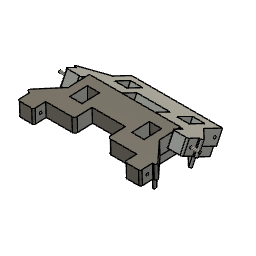
trackcomponent (Autodesk Fusion 360 design; units mm, degrees)
Autodesk Fusion 360 part; units mm, degrees
note: some values were not read from the file. Set by a fixed rule: which sketch regions a step uses.
sketch "Sketch1" plane through (0, 0, 0) normal (0, 0, 1) x (1, 0, 0)
  line L0 (0, 0) -> (0, -49.8745) construction
  line L1 (-9.5, 0) -> (-26, 0)
  line L2 (-35, 0) -> (-35, -7)
  line L3 (-35, -7) -> (-26, -7)
  line L4 (-26, -7) -> (-26, 0)
  line L5 (0, 0) -> (0, 25)
  line L6 (0, 25) -> (-26, 25)
  line L7 (-26, 25) -> (-26, 13)
  line L8 (-35, 0) -> (-38, 0)
  line L9 (-38, 0) -> (-26, 13)
  line L10 (-9.5, 0) -> (-9.5, 10)
  line L11 (-9.5, 10) -> (0, 10)
  line L12 (-21.25, 19.0231) -> (-14.25, 19.0231)
  line L13 (-14.25, 19.0231) -> (-14.25, 9.0231)
  line L14 (-14.25, 9.0231) -> (-21.25, 9.0231)
  line L15 (-21.25, 9.0231) -> (-21.25, 19.0231)
  line L16 (-36.7752, 0) -> (-25.1001, 12.6481)
  line L17 (-25.1001, 24.3) -> (-25.1001, 12.6481)
  line L18 (0, 24.3) -> (-25.1001, 24.3)
  line L19 (-34.7338, 0) -> (-23.6001, 12.0616)
  line L20 (-23.6001, 22.8) -> (-23.6001, 12.0616)
  line L21 (0, 22.8) -> (-23.6001, 22.8)
  line L22 (-34.7338, 0) -> (-35, 0)
  dimension "d1" = 35
  dimension "d3" = 9
  dimension "d8" = 7
  dimension "d10" = 25
  dimension "d12" = 3
  dimension "d13" = 10
  dimension "d14" = 10
  dimension "d15" = 7
  dimension "d19" = 12
  dimension "d20" = 9.5
  dimension "d21" = 16.5
  dimension "d22" = 4.75
  dimension "d41" = 1.5
  dimension "d42" = 1.5
  dimension "d43" = 1.5
  dimension "d44" = 0.7
  constraint vertical L0
  constraint perpendicular L0 L1
  constraint perpendicular L1 L2
  constraint perpendicular L2 L3
  constraint perpendicular L1 L4
  constraint perpendicular L1 L5
  constraint perpendicular L4 L6
  constraint perpendicular L6 L7
  constraint perpendicular L2 L8
  constraint coincident L5 L11.end
  constraint perpendicular L5 L11
  constraint horizontal L12
  constraint vertical L13
  constraint horizontal L14
  constraint vertical L15
  constraint parallel L9 L19
  constraint parallel L7 L20
  constraint parallel L6 L21
  constraint coincident L8 L19.start
  constraint parallel L9 L16
  constraint parallel L7 L17
  constraint parallel L6 L18
  constraint coincident L8 L16.start
  constraint perpendicular L2 L22
  measures "d1" distance of L0.start L2.start
  measures "d3" distance of L2.end L3.end
  measures "d8" distance of L2.start L2.end
  measures "d10" distance of L0.start L5.end
  measures "d12" distance of L2.start L8.end
  measures "d13" distance of L1.start L10.end
  measures "d14" distance of L12.start L14.end
  measures "d15" distance of L12.start L12.end
  measures "d19" distance of L6.end L7.end
  measures "d20" distance of L10.end L11.end
  measures "d21" horizontal distance of L7.end L10.end
  measures "d22" distance of L7 L15
  measures "d41" distance of L18 L21
  measures "d42" distance of L16 L19
  measures "d43" distance of L17 L20
  measures "d44" distance of L6 L18
extrude "Extrude1" add sketch "Sketch1" along normal blind 8 makes body 1
extrude "Extrude2" add sketch "Sketch1" against normal blind 5 contours L5 L8 L16 L17 L18 L19 L20 L21 L22 bodies 1
fillet "Fillet1" radius 1 2 edges at (-36.7752, 0, -2.5) (-38, 0, 4) on bodies 1
fillet "Fillet3" radius 1 2 edges at (-35, -7, 4) (-26, -7, 4) on bodies 1
fillet "Fillet4" radius 1.5 1 edges at (-9.5, 0, 4) on bodies 1
mirror "Mirror1" about plane through (0, 0, 0) normal (1, 0, 0) of bodies 1 merged
sketch "Sketch2" plane through (0, 0, 0) normal (0, 0, 1) x (1, 0, 0)
sketch "Sketch3" plane through (35, 0, 0) normal (1, 0, 0) x (0, 0, -1)
  line L0 (-8, -6) -> (0, -6)
  line L1 (0, -6) -> (0, 0)
  line L2 (0, 0) -> (-8, 0)
  line L3 (-8, 0) -> (-8, -6)
  line L4 (-8, 0) -> (0, 0)
  line L5 (0, 0) -> (0, -6)
  line L6 (0, -6) -> (-8, -6)
  line L7 (-8, -6) -> (-8, 0)
  circle A0 centre (-4, -3) radius 0.75
  dimension "d46" = 1.5
  constraint horizontal L4
  constraint vertical L5
  constraint horizontal L6
  constraint vertical L7
  constraint coincident L0.end L1.start
  constraint coincident L2.end L3.start
  measures "d46" diameter of A0
extrude "Extrude3" cut sketch "Sketch3" against normal blind 70 contours A0 bodies 1
sketch "Sketch4" plane through (-26, 0, 0) normal (-1, 0, 0) x (0, 0, 1)
  line L0 (0, 25) -> (0, 13)
  line L1 (0, 13) -> (8, 13)
  line L2 (8, 13) -> (8, 25)
  line L3 (8, 25) -> (0, 25)
  line L4 (8, 19) -> (0, 19)
  line L5 (0, 19) -> (0, 25)
  circle A0 centre (4, 22) radius 0.75
  dimension "d49" = 1.5
  constraint midpoint L2 L4.start
  constraint midpoint L0 L4.end
  constraint coincident L0.start L3.end
  measures "d49" diameter of A0
extrude "Extrude4" cut sketch "Sketch4" against normal blind 52 contours A0 bodies 1
sketch "Sketch5" plane through (0, 0, 0) normal (1, 0, 0) x (0, 0, -1)
  circle A0 centre (-33.8045, 9.7929) radius 0.75
  dimension "d52" = 1.5
  measures "d52" diameter of A0
extrude "Extrude5" add sketch "Sketch5" along normal blind 80 separate body makes body 2
copy_body "Body->Comp1" bodies 1 removing the originals makes body 3 in component "comp"
copy_body "Body->Comp2" bodies 2 removing the originals makes body 4 in component "r"
component "comp" placed x (1, 0, 0) y (0, 1, 0) z (0, 0, 1) at (51.1211, -13.5147, -10.9034)
component "r" placed x (1, 0, 0) y (0, 1, 0) z (0, 0, 1) at (11.1211, -26.3076, -40.7079)
component "comp" placed x (1, 0, 0) y (0, 1, 0) z (0, 0, 1) at (51.1211, -38.5147, -10.9034)
named bodies: "comp"
